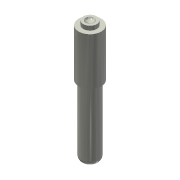
# Autodesk Inventor part: BARRA
Saved by Autodesk Inventor 2022.1 (Build 261234020, 234B)
## iProperties
Created: 2022-10-06
Part Number: BARRA
Material: Generic
Document SubType Name: Modeling
Designer: HP
Density: 1 g/cm^3
Appearance: Default
Author: HP
## iProperties of the stored document BARRA V3_3DPrint.ipt
Created: 2022-11-10
Part Number: BARRA V3_3DPrint
Material: Generic
Document SubType Name: Modeling
Designer: HP
Density: 1 g/cm^3
Appearance: Default
Author: HP
Autodesk Inventor part; units mm, degrees
ref_plane "YZ Plane" through (0, 0, 0) normal (1, 0, 0) x (0, 1, 0)
ref_plane "XZ Plane" through (0, 0, 0) normal (0, 1, 0) x (-1, 0, 0)
ref_plane "XY Plane" through (0, 0, 0) normal (0, 0, 1) x (1, 0, 0)
sketch "Sketch1" plane through (0, 0, 0) normal (0, 1, 0) x (-1, 0, 0)
  circle A0 centre (0, 0) radius 2.5
  circle A1 centre (0, 0) radius 3
  line L0 (0, 2.5) -> (0, -2.5)
  dimension "d0" = 5
  dimension "d1" = 6
  constraints: 2 centre point, 2 coincident, 2 end point, 2 point on circle, 1 vertical
  measures "d0" diameter of A0
  measures "d1" diameter of A1
extrude "Extrusion1" add sketch "Sketch1" against normal blind 15 contours A0 L0 | L0 A0 | A1
revolve "Revolution1" cut sketch "Sketch1" angle 360 about axis through (0, 0, 2.5) along (0, 0, -1) picked at (0.5196, 0.6515) contours A0 L0
sketch "Sketch2" plane through (0, 0, 0) normal (0, 1, 0) x (1, 0, 0)
  circle A0 centre (0, 0) radius 3 projected
  circle A1 centre (0, 0) radius 2.5 projected
extrude "Extrusion2" cut sketch "Sketch2" against normal blind 1.1 contours A0 | A1
sketch "Sketch3" plane through (0, -15, 0) normal (0, -1, 0) x (1, 0, 0)
  circle A0 centre (0, 0) radius 5
  circle A1 centre (0, 0) radius 3 projected
  dimension "d7" = 10
  constraints: 1 centre point, 1 coincident
  measures "d7" diameter of A0
extrude "Extrusion3" add sketch "Sketch3" against normal blind 10
sketch "Sketch4" plane through (0, -15, 0) normal (0, -1, 0) x (1, 0, 0)
  circle A0 centre (0, 0) radius 5 projected
extrude "Extrusion4" cut sketch "Sketch4" against normal blind 5
sketch "Sketch5" plane through (0, -10, 0) normal (0, -1, 0) x (1, 0, 0)
  circle A0 centre (0, 0) radius 3.95
  dimension "d12" = 7.9
  constraints: 1 centre point, 1 coincident
  measures "d12" diameter of A0
extrude "Extrusion5" add sketch "Sketch5" along normal blind 45
sketch "Sketch6" plane through (0, -5, 0) normal (0, 1, 0) x (1, 0, 0)
  circle A0 centre (0, 0) radius 3 projected
  circle A1 centre (0, 0) radius 5 projected
extrude "Extrusion6" cut sketch "Sketch6" against normal blind 0.1
sketch "Sketch7" plane through (0, -10, 0) normal (0, -1, 0) x (1, 0, 0)
  circle A0 centre (0, 0) radius 5 projected
  circle A1 centre (0, 0) radius 3.95 projected
extrude "Extrusion7" add sketch "Sketch7" along normal blind 0.1
sketch "Sketch8" plane through (0, -55, 0) normal (0, -1, 0) x (1, 0, 0)
  circle A0 centre (0, 0) radius 3.95 projected
extrude "Extrusion8" add sketch "Sketch8" along normal blind 0.1
sketch "Sketch9" plane through (0, -5.1, 0) normal (0, 1, 0) x (1, 0, 0)
  circle A0 centre (0, 0) radius 5 projected
extrude "Extrusion9" add sketch "Sketch9" along normal blind 2
sketch "Sketch10" plane through (0, -10.1, 0) normal (0, -1, 0) x (1, 0, 0)
  circle A0 centre (0, 0) radius 5 projected
  circle A1 centre (0, 0) radius 3.95 projected
extrude "Extrusion10" cut sketch "Sketch10" against normal blind 2
extrude "Extrusion11" add sketch "Sketch10" against normal blind 2
extrude "Extrusion12" add sketch "Sketch10" along normal blind 14.7
sketch "Sketch11" plane through (0, -1.1, 0) normal (0, 1, 0) x (1, 0, 0)
  circle A0 centre (0, 0) radius 3 projected
extrude "Extrusion13" cut sketch "Sketch11" against normal blind 0.3
sketch "Sketch12" plane through (0, -3.1, 0) normal (0, 1, 0) x (1, 0, 0)
  circle A0 centre (0, 0) radius 5 projected
  circle A1 centre (0, 0) radius 3 projected
extrude "Extrusion14" cut sketch "Sketch12" against normal blind 0.35
sketch "Sketch13" plane through (0, -24.8, 0) normal (0, -1, 0) x (1, 0, 0)
  circle A0 centre (0, 0) radius 3.95 projected
  circle A1 centre (0, 0) radius 5 projected
extrude "Extrusion15" cut sketch "Sketch13" against normal blind 0.35
sketch "Sketch14" plane through (0, -1.4, 0) normal (0, 1, 0) x (1, 0, 0)
  circle A0 centre (0, 0) radius 2.0712 projected
  circle A1 centre (0, 0) radius 3 projected
extrude "Extrusion16" cut sketch "Sketch14" against normal blind 0.2 contours A0 | A1
fillet "Fillet1" radius 2 1 edges at (-3.95, -55.1, 0)
body "Solid1"
